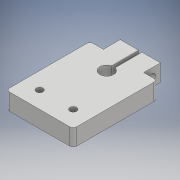
# Autodesk Inventor part: ガイド輪マウント
Saved by Autodesk Inventor 2017 (Build 210142000, 142)
## iProperties
Part Number: ガイド輪マウント
Material: 一般
Document SubType Name: Modeling
Designer: highs
Density: 1 g/cm^3
Appearance: 既定
Author: highs
## iProperties of the stored document ガイド輪マウント_3D プリント.ipt
Part Number: ガイド輪マウント_3D プリント
Material: 一般
Document SubType Name: Modeling
Designer: highs
Density: 1 g/cm^3
Appearance: 既定
Author: highs
Autodesk Inventor part; units mm, degrees
ref_plane "YZ Plane" through (0, 0, 0) normal (1, 0, 0) x (0, 1, 0)
ref_plane "XZ Plane" through (0, 0, 0) normal (0, 1, 0) x (-1, 0, 0)
ref_plane "XY Plane" through (0, 0, 0) normal (0, 0, 1) x (1, 0, 0)
sketch "スケッチ1" plane through (0, 0, 0) normal (0, 0, 1) x (1, 0, 0)
  line L0 (0, 0) -> (40, 0)
  line L1 (40, 0) -> (40, 60)
  line L2 (40, 60) -> (0, 60)
  line L3 (0, 60) -> (0, 0)
  line L4 (0, 10) -> (40, 10) construction
  circle A0 centre (10, 10) radius 2
  circle A1 centre (30, 10) radius 2
  line L5 (20, 60) -> (20, 40) construction
  circle A2 centre (20, 40) radius 4.1
  dimension "d0" = 10
  dimension "d1" = 10
  dimension "d2" = 10
  dimension "d3" = 40
  dimension "d4" = 4
  dimension "d5" = 8.2
  dimension "d6" = 40
  dimension "d7" = 20
  constraints: 12 end point, 4 perpendicular, 4 point on line, 3 centre point, 1 coincident, 1 equal radius, 1 horizontal, 1 midpoint, 1 vertical
  measures "d0" distance from line of L3 A0.centre
  measures "d1" distance between parallel lines of L0 L4
  measures "d2" distance from line of L1 A1.centre
  measures "d3" distance of L0.start L0.end
  measures "d4" diameter of A0
  measures "d5" diameter of A2
  measures "d6" distance from line of L0 L5.end
  measures "d7" distance from line of L5.end L2
extrude "押し出し1" add sketch "スケッチ1" along normal blind 10
sketch "スケッチ2" plane through (0, 0, 10) normal (0, 0, 1) x (1, 0, 0)
  line L0 (40, 60) -> (0, 60) construction
  line L1 (20, 60) -> (20, 0) construction
  line L2 (0, 0) -> (40, 0) construction
  line L3 (0, 60) -> (8, 60)
  line L4 (8, 60) -> (8, 50)
  line L5 (8, 50) -> (0, 50)
  line L6 (0, 50) -> (0, 60)
  line L7 (40, 0) -> (40, 60) projected
  line L8 (40, 60) -> (32, 60)
  line L9 (32, 60) -> (32, 50)
  line L10 (32, 50) -> (40, 50)
  line L11 (40, 50) -> (40, 60)
  line L12 (19, 80) -> (21, 80)
  line L13 (21, 80) -> (21, 40)
  line L14 (21, 40) -> (19, 40)
  line L15 (19, 40) -> (19, 80)
  line L16 (19, 80) -> (21, 40) construction
  line L17 (21, 80) -> (19, 40) construction
  circle A0 centre (20, 40) radius 4.1 projected
  dimension "d11" = 10
  dimension "d12" = 8
  dimension "d13" = 2
  constraints: 30 end point, 6 parallel, 5 midpoint, 3 horizontal, 3 perpendicular, 2 equal length, 1 coincident
  measures "d11" distance of L8.end L9.end
  measures "d12" distance of L9.end L10.end
  measures "d13" distance between parallel lines of L13 L15
extrude "押し出し2" cut sketch "スケッチ2" against normal blind 10 contours L3 L4 L5 L6 | L10 L9 L8 L7 | L12 L13 A0 L15 | A0 L13 L14 L15 picked at (19.8879, 41.3621)
sketch "スケッチ3" plane through (0, 0, 0) normal (-1, 0, 0) x (0, 0, 1)
  line L0 (0, 0) -> (10, 0) construction
  line L1 (5, 0) -> (5, 59.7235) construction
  circle A0 centre (5, 55) radius 2
  line L2 (10, 60) -> (0, 60) construction
  dimension "d16" = 5
  dimension "d17" = 4
  constraints: 2 end point, 1 centre point, 1 midpoint, 1 point on line, 1 vertical
  measures "d16" distance from line of L2 A0.centre
  measures "d17" diameter of A0
extrude "押し出し3" cut sketch "スケッチ3" against normal through all
fillet "フィレット1" radius 2 4 edges at (0, 0, 5) (40, 0, 5) (40, 50, 5) (0, 50, 5)
